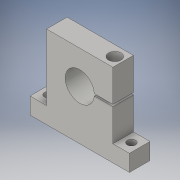
# Autodesk Inventor part: Figure 6_16_W
Saved by Autodesk Inventor 2016 (Build 200138000, 138)
## iProperties
Created: 2016-07-20
Part Number: Figure 6_16_W
Material: Generic
Document SubType Name: Modeling
Designer: cfkguest
Density: 1 g/cm^3
Appearance: Default
Author: cfkguest
Autodesk Inventor part; units mm, degrees
ref_plane "YZ Plane" through (0, 0, 0) normal (1, 0, 0) x (0, 1, 0)
ref_plane "XZ Plane" through (0, 0, 0) normal (0, 1, 0) x (-1, 0, 0)
ref_plane "XY Plane" through (0, 0, 0) normal (0, 0, 1) x (1, 0, 0)
sketch "Sketch1" plane through (0, 0, 0) normal (0, 0, 1) x (1, 0, 0)
  line L0 (0, 0) -> (76.2, 0)
  line L1 (76.2, 0) -> (76.2, 12.7)
  line L2 (76.2, 12.7) -> (63.5, 12.7)
  line L3 (63.5, 12.7) -> (63.5, 63.5)
  line L4 (63.5, 63.5) -> (12.7, 63.5)
  line L5 (12.7, 63.5) -> (12.7, 12.7)
  line L6 (12.7, 12.7) -> (0, 12.7)
  line L7 (0, 12.7) -> (0, 0)
  dimension "d0" = 12.7
  dimension "d1" = 12.7
  dimension "d2" = 76.2
  dimension "d3" = 50.8
  dimension "d4" = 12.7
  constraints: 16 end point, 6 perpendicular, 2 horizontal, 1 point on line
  measures "d0" distance of L5.end L6.end
  measures "d1" distance of L1.end L2.end
  measures "d2" distance of L0.start L0.end
  measures "d3" distance of L4.end L5.end
  measures "d4" distance of L0.end L1.end
extrude "Extrusion1" add sketch "Sketch1" along normal blind 15.748
sketch "Sketch2" plane through (0, 0, 15.748) normal (0, 0, 1) x (1, 0, 0)
  arc A0 (49.25, 38.862) -> (49.25, 37.338) centre (38.1, 38.1) ccw
  line L0 (12.7, 63.5) -> (12.7, 12.7) projected
  line L1 (63.5, 63.5) -> (12.7, 63.5) projected
  line L2 (63.5, 38.862) -> (49.25, 38.862)
  line L3 (49.25, 37.338) -> (63.5, 37.338)
  line L4 (63.5, 12.7) -> (63.5, 63.5) projected
  line L5 (63.5, 38.862) -> (63.5, 37.338)
  point P0 (0, 0)
  dimension "d7" = 22.352
  dimension "d8" = 25.4
  dimension "d9" = 25.4
  dimension "d10" = 1.524
  dimension "d11" = 24.638
  constraints: 6 end point, 2 horizontal, 2 point on circle, 1 centre point, 1 collinear, 1 point on line
  measures "d7" diameter of A0
  measures "d8" distance from line of A0.centre L0
  measures "d9" distance from line of A0.centre L1
  measures "d10" distance between parallel lines of L3 L2
  measures "d11" distance between parallel lines of L1 L2
extrude "Extrusion2" cut sketch "Sketch2" against normal blind 15.748
sketch "Sketch3" plane through (63.5, 12.7, 0) normal (0, 1, 0) x (1, 0, 0)
  line L0 (-50.8, -15.748) -> (-63.5, -15.748) projected
  line L1 (-63.5, 0) -> (-63.5, -15.748) projected
  line L2 (12.7, 0) -> (12.7, -15.748) projected
  line L3 (12.7, -15.748) -> (0, -15.748) projected
  point P0 (-57.15, -7.874)
  point P1 (6.35, -7.874)
  dimension "d14" = 7.874
  dimension "d15" = 6.35
  dimension "d16" = 6.35
  dimension "d17" = 7.874
  measures "d14" distance from line of L0 point (-57.15, -7.874)
  measures "d15" distance from line of L1 point (-57.15, -7.874)
  measures "d16" distance from line of L2 point (6.35, -7.874)
  measures "d17" distance from line of L3 point (6.35, -7.874)
hole "Hole1" at (6.35, 12.7, 7.874) at (69.85, 12.7, 7.874) direction (0, -1, 0) diameter 6.35 end through all
sketch "Sketch4" plane through (12.7, 63.5, 0) normal (0, 1, 0) x (1, 0, 0)
  line L0 (50.8, 0) -> (0, 0) projected
  line L1 (50.8, 0) -> (50.8, -15.748) projected
  point P0 (-12.7, 0)
  point P1 (44.45, -7.874)
  dimension "d25" = 7.874
  dimension "d26" = 6.35
  measures "d25" distance from line of L0 point (44.45, -7.874)
  measures "d26" distance from line of L1 point (44.45, -7.874)
hole "Hole2" at (57.15, 63.5, 7.874) direction (0, -1, 0) diameter 6.35 end through all counterbore diameter 9.652 counterbore depth 7.874
body "Solid1"
